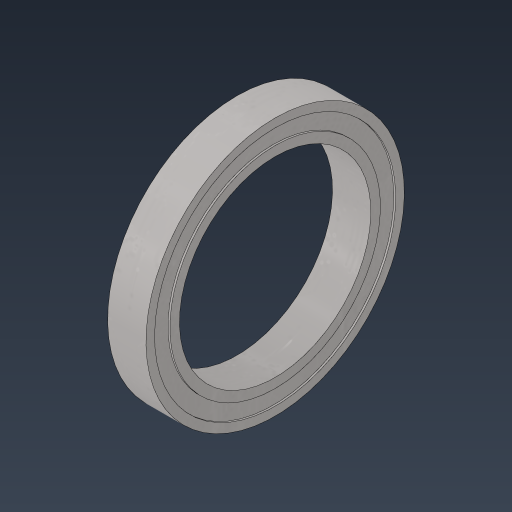
# Autodesk Inventor part: Kugellager 6704-ZZ
Saved by Autodesk Inventor 2023.1 (Build 271208000, 208)
## iProperties
Part Number: Kugellager 6704-ZZ
Material: Stahl, weich, geschweißt
Document SubType Name: Modeling
Designer: rYan
Mass: 2.82019 g
Surface Area: 4.22984 cm^2
Volume: 0.35926 cm^3
Density: 7.85 g/cm^3
Appearance: Schweißnaht - Stahl - weich
Author: rYan
Autodesk Inventor part; units mm, degrees
ref_plane "YZ Plane" through (0, 0, 0) normal (1, 0, 0) x (0, 1, 0)
ref_plane "XZ Plane" through (0, 0, 0) normal (0, 1, 0) x (-1, 0, 0)
ref_plane "XY Plane" through (0, 0, 0) normal (0, 0, 1) x (1, 0, 0)
sketch "Skizze1" plane through (0, 0, 0) normal (0, 1, 0) x (-1, 0, 0)
  line L0 (2, 0) -> (-2, 0)
  line L1 (2, 10) -> (-2, 10)
  line L2 (-2, 10) -> (-2, 11)
  line L3 (-2, 11) -> (-1.8, 11)
  line L4 (-1.8, 11) -> (-1.8, 12.6)
  line L5 (-1.8, 12.6) -> (-2, 12.6)
  line L6 (-2, 12.6) -> (-2, 13.5)
  line L7 (-2, 13.5) -> (2, 13.5)
  line L8 (2, 13.5) -> (2, 12.6)
  line L9 (2, 12.6) -> (1.8, 12.6)
  line L10 (1.8, 12.6) -> (1.8, 11)
  line L11 (1.8, 11) -> (2, 11)
  line L12 (2, 10) -> (2, 11)
  line L13 (0, -2.7) -> (0, 16.2) projected
  point P0 (0, 0)
  dimension "d0" = 20
  dimension "d1" = 27
  dimension "d2" = 4
  dimension "d3" = 0.2
  dimension "d4" = 1
  dimension "d5" = 0.9
  constraints: 26 end point, 9 point on line, 6 perpendicular, 2 vertical, 1 horizontal, 1 midpoint, 1 parallel, 4 other
  measures "d1" diameter of L7 L0
  measures "d2" distance of L6.end L7.end
  measures "d3" distance of L4.end L5.end
  measures "d4" distance of L1.end L2.end
  measures "d5" distance of L5.end L6.end
revolve "Umdrehung1" add sketch "Skizze1" angle 360 about axis through (-2, 0, 0) along (1, 0, 0)
